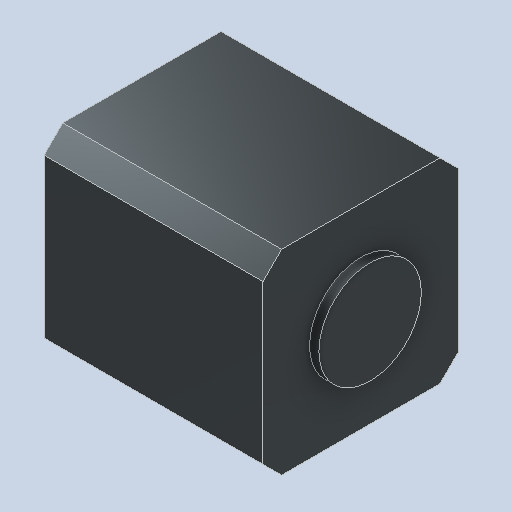
# Autodesk Inventor part: stepper
Saved by Autodesk Inventor 2023 (Build 270158000, 158)
## iProperties
Created: 2022-10-02
Part Number: stepper
Material: Iron, Cast
Document SubType Name: Modeling
Designer: carso
Density: 7.15 g/cm^3
Appearance: Iron Gray
Author: carso
Autodesk Inventor part; units mm, degrees
ref_plane "YZ Plane" through (0, 0, 0) normal (1, 0, 0) x (0, 1, 0)
ref_plane "XZ Plane" through (0, 0, 0) normal (0, 1, 0) x (-1, 0, 0)
ref_plane "XY Plane" through (0, 0, 0) normal (0, 0, 1) x (1, 0, 0)
sketch "Sketch1" plane through (0, 0, 0) normal (1, 0, 0) x (0, 1, 0)
  line L0 (-21, 21) -> (21, 21)
  line L1 (21, 21) -> (21, -21)
  line L2 (21, -21) -> (-21, -21)
  line L3 (-21, -21) -> (-21, 21)
  line L4 (-21, 21) -> (21, -21) construction
  line L5 (21, 21) -> (-21, -21) construction
  line L6 (17, 21) -> (21, 17)
  line L7 (21, 0) -> (-21, 0)
  line L8 (0, 21) -> (0, -21)
  line L9 (17, -21) -> (21, -17)
  line L10 (-17, 21) -> (-21, 17)
  line L11 (-17, -21) -> (-21, -17)
  point P0 (0, 0)
  dimension "d0" = 42
  dimension "d1" = 42
  dimension "d2" = 4
  dimension "d3" = 4
  constraints: 24 end point, 6 midpoint, 6 symmetric about line, 2 parallel, 2 point on line, 1 horizontal, 1 perpendicular
  measures "d0" distance of L1.end L2.end
  measures "d1" distance between parallel lines of L2 L0
  measures "d2" distance of L0.end L6.end
  measures "d3" distance of L0.end L6.start
extrude "Extrusion1" add sketch "Sketch1" along normal blind 47 contours L0 L8 L7 L3 L10 | L0 L6 L1 L7 L8 | L7 L8 L2 L11 L3 | L7 L1 L9 L2 L8
sketch "Sketch2" plane through (47, 0, 0) normal (1, 0, 0) x (0, 0, -1)
  circle A0 centre (0, 0) radius 11
  dimension "d6" = 22
  constraints: 1 centre point, 1 coincident
  measures "d6" diameter of A0
extrude "Extrusion2" add sketch "Sketch2" along normal blind 2
body "Solid1"
